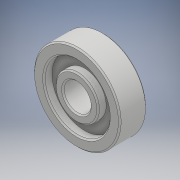
# Autodesk Inventor part: 625zz
Saved by Autodesk Inventor 2019 (Build 230136000, 136)
## iProperties
Created: 2016-04-09
Part Number: 625zz
Material: Типовые
Document SubType Name: Modeling
Designer: Admin
Density: 1 g/cm^3
Appearance: По умолчанию
Mass: 0.710589 g
Surface Area: 8.43491 cm^2
Volume: 0.710589 cm^3
Author: Admin
Autodesk Inventor part; units mm, degrees
ref_plane "YZ Plane" through (0, 0, 0) normal (1, 0, 0) x (0, 1, 0)
ref_plane "XZ Plane" through (0, 0, 0) normal (0, 1, 0) x (-1, 0, 0)
sketch "Эскиз1" plane through (0, 0, 0) normal (0, 1, 0) x (-1, 0, 0)
  circle A0 centre (0, 0) radius 8
  circle A1 centre (0, 0) radius 2.5
  circle A2 centre (0, 0) radius 4
  circle A3 centre (0, 0) radius 6
  dimension "d0" = 16
  dimension "d1" = 5
  dimension "d2" = 8
  dimension "d3" = 12
  constraints: 4 centre point, 4 coincident
  measures "d0" diameter of A0
  measures "d1" diameter of A1
  measures "d2" diameter of A2
  measures "d3" diameter of A3
extrude "Выдавливание1" add sketch "Эскиз1" along normal blind 5
chamfer "Фаска1" distance 0.25 angle 45 8 edges at (8, 0, 0) (8, 5, 0) (6, 5, 0) (2.5, 0, 0) (2.5, 5, 0) (4, 5, 0) (4, 0, 0) (6, 0, 0)
ref_plane "РабПлоскость1" through (0, 1.5, 0) normal (0, -1, 0) x (1, 0, 0)
sketch "Эскиз2" plane through (0, 1.5, 0) normal (0, -1, 0) x (1, 0, 0)
  circle A0 centre (0, 0) radius 6.25 projected
  circle A1 centre (0, 0) radius 6.7619
  circle A2 centre (0, 0) radius 3.4801
  constraints: 2 centre point, 2 coincident
extrude "Выдавливание2" add sketch "Эскиз2" against normal blind 2 contours A0
